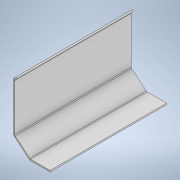
# Autodesk Inventor part: Frontal
Saved by Autodesk Inventor 2021 (Build 250183000, 183)
## iProperties
Created: 2021-07-21
Part Number: Frontal
Material: Generic
Document SubType Name: Sheet Metal
Designer: admin
Density: 1 g/cm^3
Sheet Metal Rule: Por defecto_mm
Appearance: Default
Flat Pattern Width: 32.5 cm
Flat Pattern Length: 41 cm
Flat Pattern Area: 1332.5 cm^2
Sheet Metal Width: 0.325 m
Sheet Metal Length: 0.410 m
Sheet Metal Area: 0.133 m^2
Author: admin
Autodesk Inventor part; units mm, degrees
ref_plane "YZ Plane" through (0, 0, 0) normal (1, 0, 0) x (0, 1, 0)
ref_plane "XZ Plane" through (0, 0, 0) normal (0, 1, 0) x (-1, 0, 0)
ref_plane "XY Plane" through (0, 0, 0) normal (0, 0, 1) x (1, 0, 0)
sketch "Boceto1" plane through (0, 0, 0) normal (0, 1, 0) x (-1, 0, 0)
  line L0 (162.5, 205) -> (-162.5, 205)
  line L1 (-162.5, 205) -> (-162.5, -205)
  line L2 (-162.5, -205) -> (162.5, -205)
  line L3 (162.5, -205) -> (162.5, 205)
  line L4 (162.5, 205) -> (-162.5, -205) construction
  line L5 (-162.5, 205) -> (162.5, -205) construction
  point P0 (0, 0)
  dimension "d0" = 325
  dimension "d1" = 410
  measures "d0" distance of L2.end L1.end
  measures "d1" distance of L1.end L0.end
extrude "Placa1" add sketch "Boceto1" along normal blind 5
sketch "Boceto2" plane through (0, 5, 0) normal (0, 1, 0) x (1, 0, 0)
  line L0 (-162.5, -205) -> (162.5, -205) projected
  line L1 (162.5, -205) -> (91.5, -205)
  line L2 (91.5, -205) -> (19.5, -205)
  line L3 (19.5, -205) -> (-150.5, -205)
  line L4 (91.5, -205) -> (91.5, 205) construction
  line L5 (162.5, 205) -> (-162.5, 205) construction
  line L6 (19.5, -205) -> (19.5, 205) construction
  line L7 (-150.5, -205) -> (-150.5, 205) construction
  point P0 (0, 0)
  dimension "d3" = 71
  dimension "d4" = 72
  dimension "d5" = 170
  constraints: 12 end point, 5 point on line, 2 vertical, 1 perpendicular
  measures "d3" distance of L0.end L1.end
  measures "d4" distance of L1.end L2.end
  measures "d5" distance of L2.end L3.end
fold "Pliegue1" angle 45 bend radius 5 thickness 5 k factor 0.44 line from (-150.5, 5, 205) to (-150.5, 5, -205) line at bend centre moving side (-1, 0, 0) folds toward (0, 1, 0)
fold "Pliegue2" angle 50 bend radius 5 thickness 5 k factor 0.44 line from (19.5, 5, 205) to (19.5, 5, -205) line at bend centre moving side (-1, 0, 0) folds toward (0, 1, 0)
fold "Pliegue3" angle 40 bend radius 5 thickness 5 k factor 0.44 line from (91.5, 5, 205) to (91.5, 5, -205) line at bend centre moving side (-1, 0, 0) folds toward (0, 1, 0)
equation "\"d2\" = Thickness"
equation "\"d6\" = BendReliefWidth"
equation "\"d7\" = BendReliefDepth"
equation "\"d8\" = MinimumRemnant"
equation "\"d9\" = TransitionRadius"
equation "\"d11\" = BendRadius"
equation "\"d12\" = BendReliefWidth"
equation "\"d13\" = BendReliefDepth"
equation "\"d14\" = MinimumRemnant"
equation "\"d15\" = TransitionRadius"
equation "\"d17\" = BendRadius"
equation "\"d18\" = BendReliefWidth"
equation "\"d19\" = BendReliefDepth"
equation "\"d20\" = MinimumRemnant"
equation "\"d21\" = TransitionRadius"
equation "\"d23\" = BendRadius"
equation "\"BendRadius\" = Thickness"
equation "\"BendReliefWidth\" = Thickness"
equation "\"BendReliefDepth\" = 0.5 * Thickness"
equation "\"TransitionRadius\" = BendRadius"
equation "\"JacobiRadiusSize\" = BendRadius"
equation "\"GapSize\" = Thickness"
equation "\"Thickness\" = 5"
equation "\"MinimumRemnant\" = 10"
